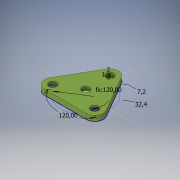
# Autodesk Inventor part: Rotor
Saved by Autodesk Inventor 2018.3 (Build 223284000, 284)
## iProperties
Created: 2018-07-20
Part Number: Rotor
Material: Generisch
Document SubType Name: Modeling
Designer: JochenAlt
Density: 1 g/cm^3
Appearance: Olivgrün
Author: JochenAlt
Autodesk Inventor part; units mm, degrees
ref_plane "YZ Plane" through (0, 0, 0) normal (1, 0, 0) x (0, 1, 0)
ref_plane "XZ Plane" through (0, 0, 0) normal (0, 1, 0) x (-1, 0, 0)
ref_plane "XY Plane" through (0, 0, 0) normal (0, 0, 1) x (1, 0, 0)
sketch "Skizze1" plane through (0, 0, 0) normal (0, 0, 1) x (1, 0, 0)
  line L0 (-29.8259, 0) -> (29.8259, 0) construction
  circle A0 centre (0, 0) radius 16.2 construction
  circle A1 centre (0, 16.2) radius 3.6
  circle A2 centre (14.0296, -8.1) radius 3.6
  circle A3 centre (-14.0296, -8.1) radius 3.6
  line L1 (0, 0) -> (-14.0296, -8.1) construction
  line L2 (0, 0) -> (14.0296, -8.1) construction
  circle A4 centre (0, 0) radius 3.6
  circle A5 centre (0, 16.2) radius 2.6
  circle A6 centre (-14.0296, -8.1) radius 2.6
  circle A7 centre (14.0296, -8.1) radius 2.6
  circle A8 centre (0, 0) radius 2.6
  arc A9 (4.8497, 19) -> (-4.8497, 19) centre (0, 16.2) ccw
  arc A10 (-18.8794, -5.3) -> (-14.0296, -13.7) centre (-14.0296, -8.1) ccw
  line L3 (14.0296, -13.7) -> (-14.0296, -13.7)
  line L4 (-18.8794, -5.3) -> (-4.8497, 19)
  line L5 (18.8794, -5.3) -> (4.8497, 19)
  arc A11 (14.0296, -13.7) -> (18.8794, -5.3) centre (14.0296, -8.1) ccw
  line L6 (0, 29.4) -> (0, -23.8) construction
  line L7 (0, 0) -> (0, 16.2) construction
  dimension "d0" = 7.2
  dimension "d1" = 32.4
  dimension "d2" = 120
  dimension "d8" = 1
  dimension "d12" = 2
  dimension "d13" = 120
  constraints: 12 centre point, 12 end point, 10 point on circle, 8 equal radius, 7 coincident, 6 tangent, 2 point on line, 1 concentric, 1 other
  measures "d0" diameter of A1
  measures "d1" diameter of A0
  measures "d2" angle of L2 L1
  measures "d8" radial gap between concentric circles of A1 A5
  measures "d12" radial gap between concentric circles of A9 A1
  measures "d13" angle of L7 L2
extrude "Extrusion1" add sketch "Skizze1" along normal blind 2 contours L5 A11 L3 A10 L4 A9
extrude "Extrusion3" add sketch "Skizze1" along normal blind 1.5 from surface at 2 contours A1 | A2 | A3 | A4 | L5 A11 L3 A10 L4 A9
equation "\"d13\" = d2"
